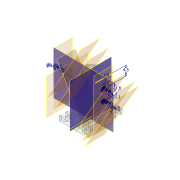
# Autodesk Inventor part: offset_cylinder
Saved by Autodesk Inventor 2021 (Build 250183000, 183)
## iProperties
Created: 2021-07-12
Part Number: offset_cylinder
Material: Generic
Document SubType Name: Modeling
Designer: Sihan
Density: 1 g/cm^3
Appearance: Default
Mass: 1.69832 g
Surface Area: 23.6767 cm^2
Volume: 1.69832 cm^3
Author: Sihan
Autodesk Inventor part; units mm, degrees
ref_plane "XZ Plane" through (0, 0, 0) normal (0, 1, 0) x (-1, 0, 0)
ref_plane "XY Plane" through (0, 0, 0) normal (0, 0, 1) x (1, 0, 0)
sketch "Sketch1" plane through (0, 0, 0) normal (0, 1, 0) x (-1, 0, 0)
  circle A0 centre (0, 0) radius 2.99
  circle A1 centre (0, 0) radius 4
  dimension "d0" = 5.98
  dimension "d1" = 8
  constraints: 2 centre point, 1 coincident
  measures "d0" diameter of A0
  measures "d1" diameter of A1
extrude "Extrusion1" add sketch "Sketch1" along normal blind 19
ref_plane "Work Plane1" through (6, 0, 0) normal (1, 0, 0) x (0, 1, 0)
sketch "Sketch2" plane through (6, 0, 0) normal (1, 0, 0) x (0, 1, 0)
  circle A0 centre (14.5, 0) radius 0.9
  circle A1 centre (9.5, 0) radius 0.9
  line L0 (19, -4) -> (19, 4) projected
  circle A2 centre (14.5, 0) radius 0.25
  circle A3 centre (9.5, 0) radius 0.25
  point P0 (0, 0)
  dimension "d5" = 1.8
  dimension "d7" = 1.8
  dimension "d9" = 4.5
  dimension "d16" = 0.5
  dimension "d18" = 0.5
  dimension "d82" = 5
  constraints: 4 centre point
  measures "d5" diameter of A0
  measures "d7" diameter of A1
  measures "d9" distance from line of L0 A0.centre
  measures "d16" diameter of A2
  measures "d18" diameter of A3
  measures "d82" distance of A1.centre A0.centre
extrude "Extrusion2" add sketch "Sketch2" against normal up to next contours A0 | A1 | A2 | A3
extrude "Extrusion3" cut sketch "Sketch2" against normal up to next contours A2 | A3
sketch "Sketch3" plane through (0, 0, 0) normal (0, 0, 1) x (1, 0, 0)
  line L0 (6, 14.75) -> (6, 14.25) projected
  line L1 (6, 14.5) -> (10.9195, 14.5)
  line L2 (6, 14.5) -> (6, 15.6)
  line L3 (6, 15.6) -> (9.5, 15.2)
  line L4 (6, 9.75) -> (6, 9.25) projected
  line L5 (6, 9.5) -> (13.6368, 9.5)
  line L6 (6, 9.5) -> (6, 10.6)
  line L7 (6, 10.6) -> (9.5, 10.2)
  line L8 (9.5, 15.2) -> (9.5, 15.05)
  line L9 (9.5, 15.05) -> (6, 15.05)
  line L10 (9.5, 10.2) -> (9.5, 10.05)
  line L11 (9.5, 10.05) -> (6, 10.05)
  point P0 (0, 0)
  point P1 (9.5, 7)
  dimension "d23" = 1.1
  dimension "d30" = 1.1
  dimension "d34" = 1.4
  dimension "d35" = 1.1
  dimension "d38" = 1.4
  dimension "d41" = 1.1
  constraints: 20 end point, 4 midpoint, 4 vertical, 2 horizontal, 2 perpendicular, 1 point on line
  measures "d23" distance of L1.start L2.end
  measures "d30" distance of L5.start L6.end
  measures "d34" diameter of L3.end L1
  measures "d35" diameter of L9 L1
  measures "d38" diameter of L7.end L5
  measures "d41" diameter of L11 L5
revolve "Revolution1" add sketch "Sketch3" angle 360 about axis through (6, 14.5, 0) along (1, 0, 0) separate body contours L2 L3 L8 L9
revolve "Revolution3" add sketch "Sketch3" angle 360 about axis through (6, 9.5, 0) along (1, 0, 0) separate body contours L6 L7 L10 L11
ref_plane "Work Plane2" through (0, 0, 0) normal (0.8660254, 0.5, 0) x (0, 0, 1)
ref_plane "Work Plane7" through (-13, 0, 0) normal (1, 0, 0) x (0, 1, 0)
sketch "Sketch4" plane through (-13, 0, 0) normal (1, 0, 0) x (0, 1, 0)
  circle A0 centre (12, 0) radius 0.9
  line L0 (19, -4) -> (19, 4) projected
  circle A1 centre (3, 0) radius 0.9
  line L1 (0, -4) -> (0, 4) projected
  point P0 (0, 0)
  dimension "d52" = 7
  dimension "d53" = 1.8
  dimension "d54" = 1.8
  dimension "d81" = 9
  constraints: 2 centre point
  measures "d52" distance from line of L0 A0.centre
  measures "d53" diameter of A0
  measures "d54" diameter of A1
  measures "d81" distance of A1.centre A0.centre
extrude "Extrusion4" add sketch "Sketch4" along normal up to next contours A0 bodies 1
sketch "Sketch5" plane through (-13, 12, 0) normal (-1, 0, 0) x (0, 0, 1)
  circle A0 centre (0, 0) radius 0.9 projected
  circle A1 centre (0, 0) radius 0.9 projected
  circle A2 centre (0, 0) radius 0.25
  circle A3 centre (0, -9) radius 0.5
  point P0 (0, -12)
  dimension "d58" = 0.5
  dimension "d59" = 1
  constraints: 2 centre point, 2 coincident
  measures "d58" diameter of A2
  measures "d59" diameter of A3
extrude "Extrusion5" cut sketch "Sketch5" against normal up to next contours A2 bodies 1
sketch "Sketch6" plane through (0, 0, 0) normal (0, 0, 1) x (1, 0, 0)
  line L0 (-13, 11.1) -> (-13, 12.9) projected
  line L1 (-13, 12) -> (-17.2091, 12)
  line L2 (-13, 12) -> (-13, 13.1)
  line L3 (-13, 13.1) -> (-16.5, 12.7)
  line L4 (-16.5, 12.7) -> (-16.5, 12.55)
  line L5 (-16.5, 12.55) -> (-13, 12.55)
  line L6 (-11, 2.1) -> (-11, 3.9) projected
  point P0 (0, 0)
  dimension "d62" = 1.1
  dimension "d63" = 1.4
  dimension "d64" = 1.1
  dimension "d138" = 3.5
  constraints: 10 end point, 2 midpoint, 2 vertical, 1 horizontal, 1 perpendicular
  measures "d62" diameter of L5 L1
  measures "d63" diameter of L3.end L1
  measures "d64" distance of L1.start L2.end
  measures "d138" horizontal distance of L2.end L3.end
revolve "Revolution5" add sketch "Sketch6" angle 360 about axis through (-13, 12, 0) along (-1, 0, 0) separate body
ref_plane "Work Plane8" through (0, 0, 0) normal (0.8660254, -0.5, 0) x (0, 0, 1)
ref_plane "Work Plane9" through (-9.1799, 5.3, 0) normal (0.8660254, -0.5, 0) x (0, 0, 1)
ref_plane "Work Plane10" through (-13.077, 7.55, 0) normal (0.8660254, -0.5, 0) x (0, 0, 1)
ref_plane "Work Plane15" through (5.1962, -3, 0) normal (0.8660254, -0.5, 0) x (0, 0, 1)
split "Split8" plane through (5.1962, -3, 0) removes the side toward (0.8660254, -0.5, 0) bodies 3
ref_plane "Work Plane16" through (3.4641, -2, 0) normal (0.8660254, -0.5, 0) x (0, 0, 1)
split "Split9" plane through (3.4641, -2, 0) removes the side toward (0.8660254, -0.5, 0) bodies 2
pattern_of_nothing "Mirror1"
pattern_of_nothing "Mirror2"
sketch "Sketch12" plane through (6, 9.5, 0) normal (1, 0, 0) x (0, 0, -1)
  circle A0 centre (0, 0) radius 0.5
  circle A1 centre (0, 0) radius 0.9 projected
  circle A2 centre (0, 5) radius 0.9 projected
  circle A3 centre (0, 0) radius 0.25 projected
  circle A4 centre (0, 5) radius 0.25 projected
  circle A5 centre (0, 5) radius 0.55 projected
  circle A6 centre (0, 5) radius 1.1 projected
  circle A7 centre (0, 0) radius 0.55 projected
  circle A8 centre (0, 0) radius 1.1 projected
  point P0 (0, -9.5)
  dimension "d106" = 1
  constraints: 1 centre point
  measures "d106" diameter of A0
extrude "Extrusion9" cut sketch "Sketch12" against normal up to surface contours A0 | A3 | A4 | A5 round surface about axis through (0, 0, 0) along (0, 1, 0) radius 2.99 far side no bodies 1
pattern_of_nothing "Mirror3"
sketch "Sketch16" plane through (0, 0, 0) normal (0, -1, 0) x (1, 0, 0)
  line L0 (-4, -9) -> (4, -9)
  line L1 (4, -9) -> (4, 9)
  line L2 (4, 9) -> (-4, 9)
  line L3 (-4, 9) -> (-4, -9)
  line L4 (-4, -9) -> (4, 9) construction
  line L5 (4, -9) -> (-4, 9) construction
  circle A0 centre (0, 0) radius 4 projected
  point P0 (-4, 0)
  point P1 (4, 0)
  dimension "d123" = 8
  dimension "d124" = 18
  constraints: 12 end point, 2 midpoint, 2 parallel, 1 horizontal, 1 perpendicular
  measures "d123" distance of L1.end L2.end
  measures "d124" distance of L0.end L1.end
extrude "Extrusion13" add sketch "Sketch16" against normal blind 2 contours L3 A0 L1 L0 | L3 L2 L1 A0 bodies 1
sketch "Sketch17" plane through (4, 0, 9) normal (1, 0, 0) x (0, 0, -1)
  line L0 (18, 0) -> (18, 2) projected
  line L1 (18, 2) -> (17, 2)
  line L2 (17, 2) -> (17, 0)
  line L3 (17, 0) -> (18, 0)
  line L4 (18, 0) -> (18, 2)
  line L5 (15, 2) -> (14, 2)
  line L6 (14, 2) -> (14, 0)
  line L7 (14, 0) -> (15, 0)
  line L8 (15, 0) -> (15, 2)
  point P0 (9, 0)
  dimension "d127" = 1
  dimension "d128" = 2
  dimension "d129" = 1
  constraints: 16 end point, 4 parallel, 2 horizontal, 2 perpendicular, 2 point on line
  measures "d127" distance between parallel lines of L8 L6
  measures "d128" distance between parallel lines of L2 L8
  measures "d129" distance between parallel lines of L0 L2
extrude "Extrusion14" add sketch "Sketch17" along normal blind 2 bodies 1
mirror "Mirror4" about plane through (0, 0, 0) normal (0, 0, 1) of "Extrusion14" bodies 1
mirror "Mirror5" about plane through (0, 0, 0) normal (1, 0, 0) of "Extrusion14", "Mirror4" bodies 1
ref_plane "Work Plane21" through (-11, 0, 0) normal (1, 0, 0) x (0, 1, 0)
sketch "Sketch18" plane through (-11, 0, 0) normal (1, 0, 0) x (0, 1, 0)
  line L0 (10.5966, 0) -> (13.4034, 0) construction
  circle A0 centre (12, 0) radius 0.55 projected
  line L1 (10.5966, -1.3) -> (13.4034, -1.3)
  line L2 (13.4034, 1.3) -> (10.5966, 1.3)
  arc A1 (10.5966, 1.3) -> (10.5966, -1.3) centre (10.5966, 0) ccw
  arc A2 (13.4034, -1.3) -> (13.4034, 1.3) centre (13.4034, 0) ccw
  circle A3 centre (12, 0) radius 0.25 projected
  circle A4 centre (12, 0) radius 0.9 projected
  point P0 (0, 0)
  dimension "d140" = 1.3
  constraints: 8 end point, 4 point on circle, 4 tangent, 2 centre point, 1 horizontal, 1 midpoint, 1 parallel
  measures "d140" radius of A2
extrude "Extrusion15" add sketch "Sketch18" along normal up to surface contours A1 L2 A2 L1 round surface about axis through (0, 0, 0) along (0, 1, 0) radius 4 far side no bodies 1
sketch "Sketch19" plane through (-13, 12, 0) normal (-1, 0, 0) x (0, 0, 1)
  circle A0 centre (0, 0) radius 0.25 projected
  circle A1 centre (0, 0) radius 0.9 projected
  circle A2 centre (0, 0) radius 1.1 projected
  circle A3 centre (0, 0) radius 0.55 projected
  point P0 (0, -12)
extrude "Extrusion16" cut sketch "Sketch19" against normal up to surface contours A0 | A3 round surface about axis through (0, 0, 0) along (0, 1, 0) radius 2.99 far side no bodies 1
fillet "Fillet4" radius 0.5 3 edges at (-11, 11.1, 0) (4, 13.6, -0.0018) (4, 8.6, -0.0018)
fillet "Fillet5" radius 0.3 1 edges at (2.99, 19, 0)
combine bodies "Combine1" operation type add bodies to combine 1 2 4 3
ref_plane "Work Plane11" through (0, 0, 0) normal (1, 0, 0) x (0, 1, 0)
ref_plane "Work Plane12" through (0, 0, 0) normal (-1, 0, 0) x (0, 1, 0)
ref_plane "Work Plane13" through (0, 0, 0) normal (-1, 0, 0) x (0, 1, 0)
ref_plane "Work Plane17" through (0, 0, 0) normal (1, 0, 0) x (0, 1, 0)
ref_plane "Work Plane18" through (0, 0, 0) normal (0, 0, 1) x (1, 0, 0)
ref_plane "Work Plane19" through (0, 0, 0) normal (0, 0, -1) x (-1, 0, 0)
ref_plane "Work Plane20" through (0, 0, 0) normal (0, 0, -1) x (-1, 0, 0)
body "Solid1"
